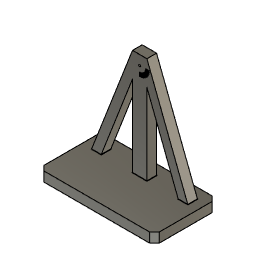
PENDULUM_V8 (Autodesk Fusion 360 design; units mm, degrees)
Autodesk Fusion 360 part; units mm, degrees
sketch "Sketch4" plane through (0, 0, 0) normal (0, 1, 0) x (1, 0, 0)
  line L0 (285, -220) -> (315, -220)
  line L1 (315, -220) -> (315, 0)
  line L2 (315, 0) -> (285, 0)
  line L3 (285, 0) -> (285, -220)
  line L4 (315, -220) -> (400, 0)
  line L5 (285, -220) -> (200, 0)
  line L6 (200, 0) -> (220, 0)
  line L7 (220, 0) -> (285, -168.2353)
  line L8 (400, 0) -> (380, 0)
  line L9 (380, 0) -> (315, -168.2353)
  line L10 (0, 0) -> (200, 0) construction
  dimension "d19" = 30
  dimension "d20" = 220
  dimension "d21" = 20
  dimension "d22" = 20
  dimension "d23" = 200
  dimension "d24" = 200
  constraint horizontal L0
  constraint vertical L1
  constraint horizontal L2
  constraint vertical L3
  constraint horizontal L6
  constraint coincident L3 L7.end
  constraint parallel L5 L7
  constraint perpendicular L1 L8
  constraint coincident L1 L9.end
  constraint parallel L4 L9
  constraint equal L4 L5
  constraint collinear L2 L8
  constraint collinear L2 L6
  constraint coincident L10.start origin
  constraint collinear L2 L10
  measures "d19" distance of L0.start L0.end
  measures "d20" distance of L0.start L2.end
  measures "d21" distance of L5.end L6.end
  measures "d22" distance of L4.end L8.end
  measures "d23" distance of L4.end L5.end
  measures "d24" distance of L5.end L10.start
extrude "Extrude4" add sketch "Sketch4" along normal blind 20 makes body 1
sketch "Sketch5" plane through (0, 0, 0) normal (0, 0, -1) x (1, 0, 0)
  line L0 (315, 0) -> (285, 0)
  line L1 (285, 0) -> (285, -20)
  line L2 (285, -20) -> (315, -20)
  line L3 (315, -20) -> (315, 0)
  line L4 (153.9541, 27.7703) -> (393.9541, 27.7703)
  line L5 (393.9541, 27.7703) -> (393.9541, 157.7703)
  line L6 (393.9541, 157.7703) -> (153.9541, 157.7703)
  line L7 (153.9541, 157.7703) -> (153.9541, 27.7703)
  line L8 (353.4541, 47.7703) -> (374.4541, 47.7703)
  line L9 (374.4541, 47.7703) -> (374.4541, 68.7703)
  line L10 (374.4541, 68.7703) -> (353.4541, 68.7703)
  line L11 (353.4541, 68.7703) -> (353.4541, 47.7703)
  line L12 (173.4541, 68.7703) -> (194.4541, 68.7703)
  line L13 (194.4541, 68.7703) -> (194.4541, 47.7703)
  line L14 (194.4541, 47.7703) -> (173.4541, 47.7703)
  line L15 (173.4541, 47.7703) -> (173.4541, 68.7703)
  line L16 (173.4541, 47.7703) -> (173.4541, 27.7703) construction
  line L17 (173.4541, 47.7703) -> (153.9541, 47.7703) construction
  line L18 (374.4541, 47.7703) -> (393.9541, 47.7703) construction
  line L19 (374.4541, 47.7703) -> (374.4541, 27.7703) construction
  line L20 (258.4541, 47.7703) -> (289.4541, 47.7703)
  line L21 (289.4541, 47.7703) -> (289.4541, 68.7703)
  line L22 (289.4541, 68.7703) -> (258.4541, 68.7703)
  line L23 (258.4541, 68.7703) -> (258.4541, 47.7703)
  line L24 (289.4541, 68.7703) -> (353.4541, 68.7703) construction
  line L25 (258.4541, 68.7703) -> (194.4541, 68.7703) construction
  dimension "d27" = 240
  dimension "d28" = 130
  dimension "d29" = 21
  dimension "d30" = 21
  dimension "d31" = 21
  dimension "d32" = 21
  dimension "d33" = 20
  dimension "d34" = 159
  dimension "d35" = 31
  dimension "d36" = 21
  constraint horizontal L4
  constraint vertical L5
  constraint horizontal L6
  constraint vertical L7
  constraint horizontal L8
  constraint vertical L9
  constraint horizontal L10
  constraint vertical L11
  constraint horizontal L12
  constraint vertical L13
  constraint horizontal L14
  constraint vertical L15
  constraint coincident L4 L16.end
  constraint perpendicular L4 L16
  constraint coincident L7 L17.end
  constraint perpendicular L7 L17
  constraint coincident L5 L18.end
  constraint perpendicular L5 L18
  constraint coincident L4 L19.end
  constraint perpendicular L4 L19
  constraint equal L16 L19
  constraint equal L17 L18
  constraint horizontal L20
  constraint vertical L21
  constraint horizontal L22
  constraint vertical L23
  constraint collinear L10 L22
  constraint equal L24 L25
  measures "d27" distance of L4.start L4.end
  measures "d28" distance of L4.start L6.end
  measures "d29" distance of L8.start L8.end
  measures "d30" distance of L8.start L10.end
  measures "d31" distance of L12.start L12.end
  measures "d32" distance of L12.start L14.end
  measures "d33" distance of L14.end L16.end
  measures "d34" distance of L11 L13
  measures "d35" distance of L20.start L20.end
  measures "d36" distance of L20.start L22.end
extrude "Extrude7" add sketch "Sketch5" along normal blind 20 separate body contours L4 L5 L6 L7 | L8 L9 L10 L11 | L12 L13 L14 L15 | L20 L21 L22 L23 makes body 2
extrude "Extrude8" cut sketch "Sketch5" along normal blind 1 contours L8 L9 L10 L11 | L12 L13 L14 L15 | L20 L21 L22 L23 bodies 2
chamfer "Chamfer1" distance 10 angle 45 4 edges at (153.9541, -157.7703, -10) (393.9541, -157.7703, -10) (393.9541, -27.7703, -10) (153.9541, -27.7703, -10) on bodies 2
move_body "Move1" bodies 1 to x (1, 0, 0) y (0, 1, 0) z (0, 0, 1) at (-6.3169, -68.1421, -0.2556)
move_body "Move2" bodies 1 to x (1, 0, 0) y (0, 1, 0) z (0, 0, 1) at (-20, 0, 0)
sketch "Sketch7" plane through (0, -68.1421, 0) normal (0, -1, 0) x (1, 0, 0)
  line L0 (288.6831, 219.7444) -> (258.6831, 219.7444)
  line L1 (258.6831, 219.7444) -> (173.6831, -0.2556)
  line L2 (173.6831, -0.2556) -> (193.6831, -0.2556)
  line L3 (193.6831, -0.2556) -> (258.6831, 167.9797)
  line L4 (258.6831, 167.9797) -> (258.6831, -0.2556)
  line L5 (258.6831, -0.2556) -> (288.6831, -0.2556)
  line L6 (288.6831, -0.2556) -> (288.6831, 167.9797)
  line L7 (288.6831, 167.9797) -> (353.6831, -0.2556)
  line L8 (353.6831, -0.2556) -> (373.6831, -0.2556)
  line L9 (373.6831, -0.2556) -> (288.6831, 219.7444)
  circle A0 centre (273.6831, 199.7444) radius 2.05
  line L10 (273.6831, 199.7444) -> (258.6831, 219.7444) construction
  line L11 (288.6831, 219.7444) -> (273.6831, 199.7444) construction
  line L12 (273.6831, 199.7444) -> (273.6831, 179.7444) construction
  line L13 (273.6831, 199.7444) -> (293.3793, 196.2714) construction
  line L14 (273.6831, 199.7444) -> (293.6831, 199.7444) construction
  line L15 (273.6831, 199.7444) -> (292.477, 192.904) construction
  line L16 (273.6831, 199.7444) -> (293.6831, 199.7444) construction
  line L17 (273.6831, 199.7444) -> (291.0036, 189.7444) construction
  line L18 (273.6831, 199.7444) -> (293.6831, 199.7444) construction
  line L19 (273.6831, 199.7444) -> (289.004, 186.8886) construction
  line L20 (273.6831, 199.7444) -> (293.6831, 199.7444) construction
  line L21 (273.6831, 199.7444) -> (286.5389, 184.4235) construction
  line L22 (273.6831, 199.7444) -> (293.6831, 199.7444) construction
  line L23 (273.6831, 199.7444) -> (283.6831, 182.4239) construction
  line L24 (273.6831, 199.7444) -> (293.6831, 199.7444) construction
  line L25 (273.6831, 199.7444) -> (280.5235, 180.9505) construction
  line L26 (273.6831, 199.7444) -> (293.6831, 199.7444) construction
  line L27 (273.6831, 199.7444) -> (277.1561, 180.0482) construction
  line L28 (273.6831, 199.7444) -> (293.6831, 199.7444) construction
  line L29 (273.1831, 179.7444) -> (274.1831, 179.7444)
  line L30 (274.1831, 179.7444) -> (274.1831, 187.7444)
  line L31 (274.1831, 187.7444) -> (273.1831, 187.7444)
  line L32 (273.1831, 187.7444) -> (273.1831, 179.7444)
  line L33 (273.1831, 179.7444) -> (274.1831, 179.7444)
  line L34 (274.1831, 179.7444) -> (274.1831, 187.7444)
  line L35 (273.1831, 187.7444) -> (273.1831, 179.7444)
  line L36 (274.1831, 187.7444) -> (273.1831, 187.7444)
  line L37 (276.6637, 179.9614) -> (277.6485, 180.1351)
  line L38 (277.6485, 180.1351) -> (276.2593, 188.0135)
  line L39 (275.2745, 187.8399) -> (276.6637, 179.9614)
  line L40 (276.2593, 188.0135) -> (275.2745, 187.8399)
  line L41 (280.0537, 180.7795) -> (280.9934, 181.1215)
  line L42 (280.9934, 181.1215) -> (278.2572, 188.6391)
  line L43 (277.3175, 188.2971) -> (280.0537, 180.7795)
  line L44 (278.2572, 188.6391) -> (277.3175, 188.2971)
  line L45 (283.2501, 182.1739) -> (284.1162, 182.6739)
  line L46 (284.1162, 182.6739) -> (280.1162, 189.6021)
  line L47 (279.2501, 189.1021) -> (283.2501, 182.1739)
  line L48 (280.1162, 189.6021) -> (279.2501, 189.1021)
  line L49 (286.1559, 184.1021) -> (286.9219, 184.7449)
  line L50 (286.9219, 184.7449) -> (281.7796, 190.8732)
  line L51 (281.0136, 190.2305) -> (286.1559, 184.1021)
  line L52 (281.7796, 190.8732) -> (281.0136, 190.2305)
  line L53 (288.6826, 186.5056) -> (289.3254, 187.2717)
  line L54 (289.3254, 187.2717) -> (283.1971, 192.414)
  line L55 (282.5543, 191.6479) -> (288.6826, 186.5056)
  line L56 (283.1971, 192.414) -> (282.5543, 191.6479)
  line L57 (290.7536, 189.3114) -> (291.2536, 190.1774)
  line L58 (291.2536, 190.1774) -> (284.3254, 194.1774)
  line L59 (283.8254, 193.3114) -> (290.7536, 189.3114)
  line L60 (284.3254, 194.1774) -> (283.8254, 193.3114)
  line L61 (292.306, 192.4341) -> (292.648, 193.3738)
  line L62 (292.648, 193.3738) -> (285.1305, 196.11)
  line L63 (284.7884, 195.1703) -> (292.306, 192.4341)
  line L64 (285.1305, 196.11) -> (284.7884, 195.1703)
  line L65 (293.2925, 195.779) -> (293.4661, 196.7638)
  line L66 (293.4661, 196.7638) -> (285.5877, 198.153)
  line L67 (285.414, 197.1682) -> (293.2925, 195.779)
  line L68 (285.5877, 198.153) -> (285.414, 197.1682)
  line L69 (293.6831, 199.2444) -> (293.6831, 200.2444)
  line L70 (293.6831, 200.2444) -> (285.6831, 200.2444)
  line L71 (285.6831, 199.2444) -> (293.6831, 199.2444)
  line L72 (285.6831, 200.2444) -> (285.6831, 199.2444)
  dimension "d53" = 4.1
  dimension "d54" = 20
  dimension "d57" = 20
  dimension "d58" = 10
  dimension "d59" = 20
  dimension "d60" = 20
  dimension "d61" = 20
  dimension "d62" = 20
  dimension "d63" = 30
  dimension "d64" = 40
  dimension "d65" = 20
  dimension "d66" = 50
  dimension "d67" = 20
  dimension "d68" = 20
  dimension "d69" = 60
  dimension "d70" = 70
  dimension "d71" = 20
  dimension "d72" = 80
  dimension "d73" = 20
  dimension "d74" = 1
  dimension "d75" = 8
  dimension "d76" = 1
  dimension "d77" = 8
  dimension "d78" = 1
  dimension "d79" = 8
  dimension "d80" = 1
  dimension "d81" = 8
  dimension "d82" = 1
  dimension "d83" = 8
  dimension "d84" = 1
  dimension "d85" = 8
  dimension "d86" = 1
  dimension "d87" = 8
  dimension "d88" = 1
  dimension "d89" = 8
  dimension "d90" = 1
  dimension "d91" = 8
  dimension "d92" = 1
  dimension "d93" = 8
  dimension "d94" = 1
  dimension "d95" = 8
  constraint coincident A0.centre L10.start
  constraint coincident L0.end L1.start
  constraint coincident L0.start L9.end
  constraint equal L10 L11
  constraint vertical L12
  constraint horizontal L14
  constraint horizontal L16
  constraint horizontal L18
  constraint horizontal L20
  constraint horizontal L22
  constraint horizontal L24
  constraint horizontal L26
  constraint horizontal L28
  constraint horizontal L29
  constraint vertical L30
  constraint horizontal L31
  constraint vertical L32
  constraint midpoint L12.end L29
  constraint horizontal L33
  constraint vertical L34
  constraint horizontal L36
  constraint vertical L35
  constraint midpoint L27.end L37
  constraint midpoint L25.end L41
  constraint midpoint L23.end L45
  constraint midpoint L14.end L69
  constraint midpoint L13.end L65
  constraint midpoint L15.end L61
  constraint midpoint L17.end L57
  constraint midpoint L19.end L53
  constraint midpoint L21.end L49
  measures "d53" diameter of A0
  measures "d54" distance of L0 A0.centre
  measures "d57" distance of A0.centre L12.end
  measures "d58" angle of L13 L14
  measures "d59" distance of A0.centre L13.end
  measures "d60" angle of L15 L16
  measures "d61" distance of A0.centre L15.end
  measures "d62" distance of A0.centre L17.end
  measures "d63" angle of L17 L18
  measures "d64" angle of L19 L20
  measures "d65" distance of A0.centre L19.end
  measures "d66" angle of L21 L22
  measures "d67" distance of A0.centre L21.end
  measures "d68" distance of A0.centre L23.end
  measures "d69" angle of L23 L24
  measures "d70" angle of L25 L26
  measures "d71" distance of A0.centre L25.end
  measures "d72" angle of L27 L28
  measures "d73" distance of A0.centre L27.end
  measures "d74" distance of L29.start L29.end
  measures "d75" distance of L29.start L31.end
  measures "d76" distance of L29.start L29.end
  measures "d77" distance of L29.start L31.end
  measures "d78" distance of L37.start L37.end
  measures "d79" distance of L37.start L39.start
  measures "d80" distance of L41.start L41.end
  measures "d81" distance of L41.start L43.start
  measures "d82" distance of L45.start L45.end
  measures "d83" distance of L45.start L47.start
  measures "d84" distance of L49.start L49.end
  measures "d85" distance of L49.start L51.start
  measures "d86" distance of L53.start L53.end
  measures "d87" distance of L53.start L55.start
  measures "d88" distance of L57.start L57.end
  measures "d89" distance of L57.start L59.start
  measures "d90" distance of L61.start L61.end
  measures "d91" distance of L61.start L63.start
  measures "d92" distance of L65.start L65.end
  measures "d93" distance of L65.start L67.start
  measures "d94" distance of L69.start L69.end
  measures "d95" distance of L69.start L71.start
extrude "Extrude11" cut sketch "Sketch7" against normal blind 52 contours A0 bodies 1
extrude "Extrude12" cut sketch "Sketch7" against normal blind 2 contours L29 L30 L31 L32 L33 L34 L35 L36 | L37 L38 L39 L40 | L41 L42 L43 L44 | L45 L46 L47 L48 | L49 L50 L51 L52 | L53 L54 L55 L56 | L57 L58 L59 L60 | L61 L62 L63 L64 | L65 L66 L67 L68 | L69 L70 L71 L72 bodies 1
equation "d34 = 160 mm - 1 mm"
